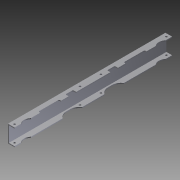
# Autodesk Inventor part: 2.25 U frame 2
Saved by Autodesk Inventor 2012 (Build 160160000, 160)
## iProperties
Created: 2013-11-06
Part Number: 2.25 U frame 2
Material: Default
Document SubType Name: Modeling
Designer: Bryce
Density: 1 g/cm^3
Author: Bryce
Autodesk Inventor part; units mm, degrees
ref_plane "YZ Plane" through (0, 0, 0) normal (1, 0, 0) x (0, 1, 0)
ref_plane "XZ Plane" through (0, 0, 0) normal (0, 1, 0) x (-1, 0, 0)
ref_plane "XY Plane" through (0, 0, 0) normal (0, 0, 1) x (1, 0, 0)
sketch "Sketch1" plane through (0, 0, 0) normal (0, 0, 1) x (1, 0, 0)
  line L0 (0, 0) -> (22.225, 0)
  line L1 (22.225, 0) -> (22.225, 57.15)
  line L2 (22.225, 57.15) -> (0, 57.15)
  line L3 (0, 57.15) -> (0, 0)
  line L4 (3.175, 3.175) -> (22.225, 3.175)
  line L5 (22.225, 3.175) -> (22.225, 53.975)
  line L6 (22.225, 53.975) -> (3.175, 53.975)
  line L7 (3.175, 53.975) -> (3.175, 3.175)
  dimension "d0" = 3.175
  dimension "d1" = 3.175
  dimension "d2" = 3.175
  dimension "d3" = 57.15
  dimension "d4" = 22.225
  constraints: 16 end point, 4 parallel, 2 horizontal, 2 perpendicular, 1 coincident, 1 point on line
  measures "d0" distance between parallel lines of L0 L4
  measures "d1" distance between parallel lines of L3 L7
  measures "d2" distance between parallel lines of L6 L2
  measures "d3" distance of L2.end L0.start
  measures "d4" distance of L0.start L0.end
extrude "Extrusion1" add sketch "Sketch1" along normal blind 527.05 contours L3 L2 L1 L6 L7 L4 L0
sketch "Sketch2" plane through (0, 57.15, 0) normal (0, 1, 0) x (1, 0, 0)
  line L0 (22.225, 0) -> (22.225, -527.05) projected
  line L1 (0, 0) -> (0, -527.05) projected
  line L2 (22.7547, 0) -> (0, 0)
  line L3 (22.225, -85.725) -> (15.875, -85.725)
  line L4 (15.875, -85.725) -> (15.875, -155.575)
  line L5 (15.875, -155.575) -> (22.225, -155.575)
  line L6 (22.225, -155.575) -> (22.225, -85.725)
  line L7 (22.225, -180.975) -> (11.43, -180.975)
  line L8 (11.43, -180.975) -> (11.43, -206.375)
  line L9 (11.43, -206.375) -> (22.225, -206.375)
  line L10 (22.225, -206.375) -> (22.225, -180.975)
  arc A0 (22.225, -21.2995) -> (22.225, -54.9005) centre (41.275, -38.1) ccw
  circle A1 centre (12.7, -9.525) radius 3.175
  circle A2 centre (12.7, -228.6) radius 3.175
  line L11 (3.175, 0) -> (3.175, -527.05) projected
  line L12 (22.225, 0) -> (0, 0) projected
  line L13 (22.225, -21.2995) -> (22.225, -54.9005)
  line L14 (0, -263.525) -> (22.225, -263.525) construction
  line L15 (22.225, -346.075) -> (11.43, -346.075)
  line L16 (11.43, -346.075) -> (11.43, -320.675)
  line L17 (22.225, -320.675) -> (22.225, -346.075)
  line L18 (11.43, -320.675) -> (22.225, -320.675)
  circle A3 centre (12.7, -298.45) radius 3.175
  line L19 (15.875, -371.475) -> (22.225, -371.475)
  line L20 (15.875, -441.325) -> (15.875, -371.475)
  line L21 (22.225, -371.475) -> (22.225, -441.325)
  line L22 (22.225, -441.325) -> (15.875, -441.325)
  arc A4 (22.225, -472.1495) -> (22.225, -505.7505) centre (41.275, -488.95) ccw
  circle A5 centre (12.7, -517.525) radius 3.175
  line L23 (22.225, -527.05) -> (0, -527.05)
  line L24 (22.225, -505.7505) -> (22.225, -472.1495)
  dimension "d7" = 85.725
  dimension "d8" = 69.85
  dimension "d9" = 6.35
  dimension "d10" = 180.975
  dimension "d11" = 25.4
  dimension "d12" = 25.4
  dimension "d13" = 38.1
  dimension "d14" = 9.525
  dimension "d15" = 6.35
  dimension "d16" = 228.6
  dimension "d17" = 38.1
  dimension "d18" = 11.43
  dimension "d21" = 263.525
  constraints: 42 end point, 13 symmetric about line, 6 centre point, 4 parallel, 4 point on circle, 3 collinear, 3 perpendicular, 2 horizontal, 2 midpoint, 2 point on line, 1 equal radius, 1 vertical alignment, 3 other
  measures "d7" distance between parallel lines of L2 L3
  measures "d8" distance of L4.start L5.start
  measures "d9" distance of L6.end L4.start
  measures "d10" distance between parallel lines of L2 L7
  measures "d11" distance between parallel lines of L9 L7
  measures "d12" radius of A0
  measures "d13" distance from line of A0.centre L2
  measures "d14" distance from line of L2 A1.centre
  measures "d15" diameter of A1
  measures "d16" distance from line of L2 A2.centre
  measures "d17" distance from line of L11 A0.centre
  measures "d18" distance between parallel lines of L1 L8
  measures "d21" distance between parallel lines of L12 L14
extrude "Extrusion2" cut sketch "Sketch2" against normal blind 3.175 contours L0 A0 | L0 L5 L4 L3 | A4 L0 | L0 L9 L8 L7 | L22 L20 L19 L0 | L0 L15 L16 L18 | A1 | A2 | A3 | A5
sketch "Sketch3" plane through (0, 0, 0) normal (0, -1, 0) x (1, 0, 0)
  line L0 (0, 0) -> (0, 527.05) projected
  line L1 (0, 0) -> (22.225, 0) projected
  line L2 (22.225, 0) -> (22.225, 527.05) projected
  line L3 (0, 0) -> (0, 301.9932)
  line L4 (0, 0) -> (22.225, 0)
  line L5 (22.225, 0) -> (22.225, 21.2995)
  arc A0 (7.9375, 187.325) -> (22.225, 160.8085) centre (39.6875, 187.325) ccw
  line L6 (7.9375, 187.325) -> (7.9375, 200.025)
  arc A1 (22.225, 226.5415) -> (7.9375, 200.025) centre (39.6875, 200.025) ccw
  arc A2 (22.225, 54.9005) -> (22.225, 21.2995) centre (41.275, 38.1) ccw
  circle A3 centre (12.7, 9.525) radius 3.175
  circle A4 centre (12.7, 228.6) radius 3.175
  line L7 (3.175, 0) -> (3.175, 527.05) projected
  line L8 (0, 263.525) -> (22.225, 263.525) construction
  line L9 (22.225, 160.8085) -> (22.225, 226.5415)
  line L10 (22.225, 226.5415) -> (22.225, 302.1048)
  line L11 (22.225, 21.2995) -> (22.225, 54.9005)
  line L12 (22.225, 54.9005) -> (22.225, 160.8085)
  arc A5 (22.225, 366.2415) -> (7.9375, 339.725) centre (39.6875, 339.725) ccw
  line L13 (7.9375, 339.725) -> (7.9375, 327.025)
  arc A6 (7.9375, 327.025) -> (22.225, 300.5085) centre (39.6875, 327.025) ccw
  arc A7 (22.225, 505.7505) -> (22.225, 472.1495) centre (41.275, 488.95) ccw
  circle A8 centre (12.7, 517.525) radius 3.175
  circle A9 centre (12.7, 298.45) radius 3.175
  line L14 (22.225, 366.2415) -> (22.225, 300.5085)
  line L15 (22.225, 505.7505) -> (22.225, 472.1495)
  dimension "d22" = 31.75
  dimension "d23" = 12.7
  dimension "d24" = 187.325
  dimension "d25" = 7.9375
  dimension "d26" = 38.1
  dimension "d27" = 38.1
  dimension "d28" = 25.4
  dimension "d29" = 263.525
  constraints: 24 end point, 12 point on circle, 11 symmetric about line, 10 centre point, 3 point on line, 2 collinear, 2 midpoint, 2 tangent, 1 equal radius, 1 perpendicular, 5 other
  measures "d22" radius of A0
  measures "d23" distance of L6.start L6.end
  measures "d24" distance from line of L4 L6.start
  measures "d25" distance between parallel lines of L6 L3
  measures "d26" distance from line of L7 A2.centre
  measures "d27" distance from line of A2.centre L1
  measures "d28" radius of A2
  measures "d29" distance from line of L1.end L8
extrude "Extrusion3" cut sketch "Sketch3" against normal blind 3.175
fillet "Fillet1" radius 3.175 8 edges at (15.875, 55.5625, 441.325) (15.875, 55.5625, 371.475) (11.43, 55.5625, 346.075) (11.43, 55.5625, 320.675) (11.43, 55.5625, 206.375) (11.43, 55.5625, 180.975) (15.875, 55.5625, 155.575) (15.875, 55.5625, 85.725)
equation "\"d1\" = d0"
equation "\"d2\" = d0"
body "Solid1"
